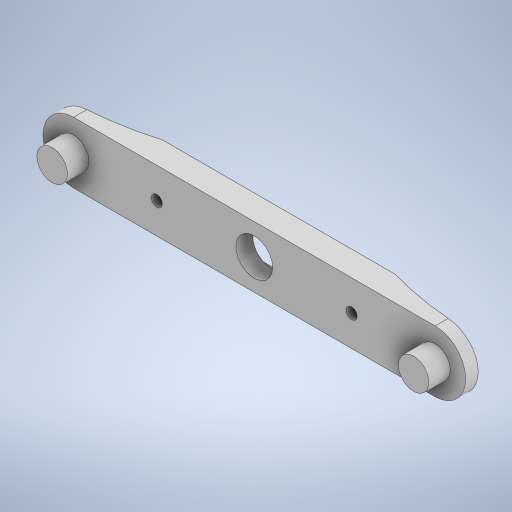
# Autodesk Inventor part: gripper_mechanism1
Saved by Autodesk Inventor 2023 (Build 270158000, 158)
## iProperties
Created: 2024-07-17
Part Number: gripper_mechanism1
Material: Generic
Document SubType Name: Modeling
Designer: Swoby
Density: 1 g/cm^3
Appearance: Default
Author: Swoby
Autodesk Inventor part; units mm, degrees
ref_plane "YZ Plane" through (0, 0, 0) normal (1, 0, 0) x (0, 1, 0)
ref_plane "XZ Plane" through (0, 0, 0) normal (0, 1, 0) x (-1, 0, 0)
ref_plane "XY Plane" through (0, 0, 0) normal (0, 0, 1) x (1, 0, 0)
sketch "Sketch1" plane through (0, 0, 0) normal (0, 0, 1) x (1, 0, 0)
  circle A0 centre (0, 0) radius 3
  circle A1 centre (0, 0) radius 5 construction
  circle A2 centre (-29.5, 0) radius 2.5
  circle A3 centre (29.5, 0) radius 2.5
  line L0 (-29.5, 0) -> (29.5, 0) construction
  arc A4 (-29.5, 5) -> (-29.5, -5) centre (-29.5, 0) ccw
  arc A5 (29.5, -5) -> (29.5, 5) centre (29.5, 0) ccw
  line L1 (-29.5, 5) -> (29.5, 5)
  line L2 (29.5, -5) -> (-29.5, -5)
  dimension "d0" = 6
  dimension "d1" = 10
  dimension "d2" = 5
  dimension "d3" = 5
  dimension "d4" = 29.5
  dimension "d5" = 29.5
  dimension "d6" = 2.5
  dimension "d7" = 2.5
  constraints: 6 centre point, 6 end point, 4 point on circle, 3 tangent, 2 coincident, 2 horizontal, 1 midpoint
  measures "d0" diameter of A0
  measures "d1" diameter of A1
  measures "d2" diameter of A2
  measures "d3" diameter of A3
  measures "d4" distance of point (0, 0) L0.start
  measures "d5" distance of point (0, 0) L0.end
  measures "d6" radial gap between concentric circles of A2 A4
  measures "d7" radial gap between concentric circles of A3 A5
extrude "Extrusion1" add sketch "Sketch1" along normal blind 4.05
sketch "Sketch2" plane through (0, 0, 0) normal (0, 0, -1) x (-1, 0, 0)
  line L0 (-5.5, -4) -> (5.5, -4)
  line L1 (5.5, -4) -> (5.5, 4)
  line L2 (5.5, 4) -> (-5.5, 4)
  line L3 (-5.5, 4) -> (-5.5, -4)
  line L4 (-5.5, -4) -> (5.5, 4) construction
  line L5 (5.5, -4) -> (-5.5, 4) construction
  line L6 (-29.5, 5) -> (29.5, 5) projected
  point P0 (0, 0)
  dimension "d10" = 8
  dimension "d11" = 11
  constraints: 12 end point, 3 parallel, 2 midpoint, 1 perpendicular
  measures "d10" distance of L0.end L1.end
  measures "d11" distance of L1.end L2.end
extrude "Extrusion2" cut sketch "Sketch2" against normal blind 1.3
sketch "Sketch3" plane through (0, 0, 0) normal (0, 0, -1) x (-1, 0, 0)
  circle A0 centre (-29.5, 0) radius 2.5 projected
  circle A1 centre (29.5, 0) radius 2.5 projected
  point P0 (0, 0)
extrude "Extrusion3" add sketch "Sketch3" against normal blind 7.55
sketch "Sketch4" plane through (-29.5, 5, 0) normal (0, 1, 0) x (1, 0, 0)
  line L0 (64, 0) -> (64, -4.05) projected
  line L1 (64, -2) -> (64, 0)
  line L2 (59, 0) -> (64, 0) projected
  line L3 (64, 0) -> (48.5, 0)
  arc A0 (48.5, 0) -> (64, -2) centre (62.5699, 47.9795) ccw
  line L4 (59, 0) -> (0, 0) projected
  line L5 (29.5, 0) -> (29.5, -4.05)
  line L6 (59, -4.05) -> (0, -4.05) projected
  line L7 (-5, -2) -> (-5, 0)
  line L8 (0, 0) -> (-5, 0)
  line L9 (-5, 0) -> (10.5, 0)
  arc A1 (-5, -2) -> (10.5, 0) centre (-3.5699, 47.9795) ccw
  dimension "d16" = 19
  dimension "d17" = 2
  dimension "d18" = 50
  constraints: 12 end point, 5 symmetric about line, 4 point on circle, 3 point on line, 2 centre point, 2 midpoint, 1 other
  measures "d16" distance of L5.start L3.end
  measures "d17" distance of L0.start L1.start
  measures "d18" radius of A0
extrude "Extrusion4" cut sketch "Sketch4" against normal through all
sketch "Sketch5" plane through (0, 0, 0) normal (0, 0, -1) x (-1, 0, 0)
  circle A0 centre (15.9, 0) radius 0.9
  circle A1 centre (-15.9, 0) radius 0.9
  line L0 (15.9, 0) -> (-15.9, 0)
  point P0 (0, 0)
  dimension "d21" = 1.8
  dimension "d22" = 1.8
  dimension "d24" = 15.9
  constraints: 2 centre point, 2 end point, 2 midpoint, 1 horizontal
  measures "d21" diameter of A0
  measures "d22" diameter of A1
  measures "d24" distance of L0.start point (0, 0)
extrude "Extrusion5" cut sketch "Sketch5" against normal through all
equation "\"d3\" = d2"
equation "\"d5\" = d4"
body "Solid1"
